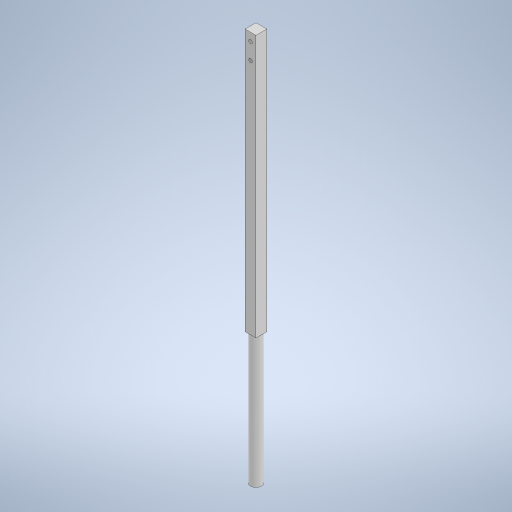
# Autodesk Inventor part: handle
Saved by Autodesk Inventor 2023 (Build 270158000, 158)
## iProperties
Created: 2023-01-06
Part Number: handle
Material: Generic
Document SubType Name: Modeling
Designer: Hayden Swanson
Density: 1 g/cm^3
Appearance: Default
Author: Hayden Swanson
Autodesk Inventor part; units mm, degrees
ref_plane "YZ Plane" through (0, 0, 0) normal (1, 0, 0) x (0, 1, 0)
ref_plane "XZ Plane" through (0, 0, 0) normal (0, 1, 0) x (-1, 0, 0)
ref_plane "XY Plane" through (0, 0, 0) normal (0, 0, 1) x (1, 0, 0)
sketch "Sketch1" plane through (0, 0, 0) normal (0, 1, 0) x (-1, 0, 0)
  line L0 (0, 0) -> (6.35, 0)
  line L1 (6.35, 0) -> (6.35, -6.35)
  line L2 (6.35, -6.35) -> (0, -6.35)
  line L3 (0, -6.35) -> (0, 0)
  dimension "d0" = 6.35
  dimension "d1" = 6.35
  constraints: 8 end point, 2 parallel, 1 horizontal, 1 perpendicular
  measures "d0" distance of L1.end L2.end
  measures "d1" distance of L0.end L1.end
extrude "Extrusion1" add sketch "Sketch1" along normal blind 152.4
sketch "Sketch3" plane through (0, 0, 0) normal (0, -1, 0) x (1, 0, 0)
  line L0 (0, 0) -> (0, -6.35) projected
  line L1 (0, 0) -> (0, -3.175)
  line L2 (0, -3.175) -> (-6.35, -3.175)
  line L3 (-6.35, -6.35) -> (-6.35, 0) projected
  line L4 (-6.35, 0) -> (0, 0) projected
  line L5 (-3.175, 0) -> (-3.175, -6.35)
  line L6 (0, -6.35) -> (-6.35, -6.35) projected
  line L7 (0, -6.35) -> (-6.35, -6.35) projected
  line L8 (0, 0) -> (0, -6.35) projected
  line L9 (-6.35, -6.35) -> (-6.35, 0) projected
  circle A0 centre (-3.175, -3.175) radius 3.175
  dimension "d12" = 6.35
  constraints: 6 end point, 5 midpoint, 1 centre point
  measures "d12" diameter of A0
extrude "Extrusion3" add sketch "Sketch3" along normal blind 76.2 contours A0 L5 L2 | L2 L5 A0 | L5 L2 A0 | L5 A0 L2
sketch "Sketch4" plane through (-6.35, 152.4, 0) normal (0, 0, 1) x (1, 0, 0)
  line L0 (6.35, 0) -> (0, 0) projected
  line L1 (3.175, 0) -> (3.175, -4.7625)
  circle A0 centre (3.175, -4.7625) radius 1.4224
  line L2 (3.175, -4.7625) -> (3.175, -14.2875)
  circle A1 centre (3.175, -14.2875) radius 1.4224
  point P0 (6.35, -152.4)
  dimension "d15" = 4.7625
  dimension "d16" = 2.8448
  dimension "d17" = 9.525
  dimension "d18" = 2.8448
  constraints: 4 end point, 2 centre point, 2 coincident, 2 vertical, 1 midpoint
  measures "d15" distance of L1.start L1.end
  measures "d16" diameter of A0
  measures "d17" distance of L2.start L2.end
  measures "d18" diameter of A1
hole "Hole1" at (-3.175, 147.6375, 0) at (-3.175, 138.1125, 0) direction (0, 0, -1) diameter 2.1565 end through all thread size "4-40 UNC" class "3B" standard "ANSI Unified Screw Threads"
body "Solid1"
